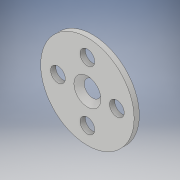
# Autodesk Inventor part: piercable_septum_clamp
Saved by Autodesk Inventor 2019.4 (Build 234330000, 330)
## iProperties
Created: 2021-04-23
Part Number: piercable_septum_clamp
Material: Generic
Document SubType Name: Modeling
Designer: PattersonOfficeMini
Density: 1 g/cm^3
Appearance: Default
Author: PattersonOfficeMini
Autodesk Inventor part; units mm, degrees
ref_plane "YZ Plane" through (0, 0, 0) normal (1, 0, 0) x (0, 1, 0)
ref_plane "XZ Plane" through (0, 0, 0) normal (0, 1, 0) x (-1, 0, 0)
ref_plane "XY Plane" through (0, 0, 0) normal (0, 0, 1) x (1, 0, 0)
sketch "Sketch1" plane through (0, 0, 0) normal (0, 0, 1) x (1, 0, 0)
  circle A0 centre (0, 0) radius 14.2875
  dimension "d0" = 28.575
  constraints: 1 centre point, 1 coincident
  measures "d0" diameter of A0
extrude "Extrusion1" add sketch "Sketch1" along normal blind 1.5875
sketch "Sketch2" plane through (0, 0, 1.5875) normal (0, 0, 1) x (1, 0, 0)
  point P0 (0, 0)
  point P1 (0, 9.017)
  point P2 (9.017, 0)
  point P3 (0, -9.017)
  point P4 (-9.017, 0)
  dimension "d3" = 9.017
  dimension "d4" = 9.017
  dimension "d5" = 9.017
  dimension "d6" = 9.017
  measures "d3" distance of point (0, 9.017) point (0, 0)
  measures "d4" distance of point (0, 0) point (9.017, 0)
  measures "d5" distance of point (0, 0) point (0, -9.017)
  measures "d6" distance of point (0, 0) point (-9.017, 0)
hole "Hole1" at (0, 9.017, 1.5875) at (9.017, 0, 1.5875) at (0, -9.017, 1.5875) at (-9.017, 0, 1.5875) direction (0, 0, -1) diameter 4.4958 depth 12.2936 tip angle 118 clearance for "Flat Head Machine Screw (82)" size "#8" standard "Ansi Unified Screw Threads"
sketch "Sketch3" plane through (0, 0, 1.5875) normal (0, 0, 1) x (1, 0, 0)
  circle A0 centre (0, 0) radius 2.54
  dimension "d14" = 5.08
  constraints: 1 centre point, 1 coincident
  measures "d14" diameter of A0
extrude "Extrusion2" cut sketch "Sketch3" against normal blind 1.5875
chamfer "Chamfer1" distance 1.5875 angle 45 1 edges at (-2.54, 0, 1.5875)
body "Solid1"
